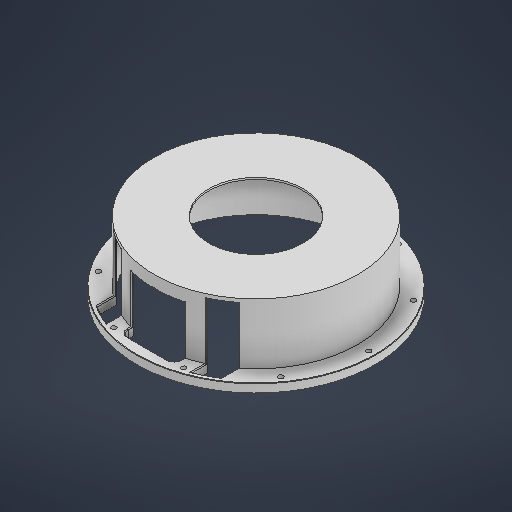
# Autodesk Inventor part: Cylinder  Segment - 01
Saved by Autodesk Inventor 2025 (Build 290162000, 162)
## iProperties
Created: 2024-04-11
Part Number: Cylinder  Segment - 01
Material: Generic
Document SubType Name: Modeling
Designer: Thienan Hoang
Density: 1 g/cm^3
Appearance: Default
Author: Thienan Hoang
Autodesk Inventor part; units mm, degrees
ref_plane "YZ Plane" through (0, 0, 0) normal (1, 0, 0) x (0, 1, 0)
ref_plane "XZ Plane" through (0, 0, 0) normal (0, 1, 0) x (-1, 0, 0)
ref_plane "XY Plane" through (0, 0, 0) normal (0, 0, 1) x (1, 0, 0)
sketch "Sketch1" plane through (0, 0, 0) normal (0, 1, 0) x (-1, 0, 0)
  circle A0 centre (0, 0) radius 135
  circle A1 centre (0, 0) radius 115
  circle A2 centre (0, 0) radius 112.0375
  circle A3 centre (0, 0) radius 9.5
  dimension "Absolute_Diameter" = 270
  dimension "Diameter_No_Outer_Lip" = 230
  dimension "Inner_Cylinder_Diameter" = 224.075
  dimension "Lip_Diameter" = 19
  constraints: 4 centre point, 4 coincident
  measures "Absolute_Diameter" diameter of A0
  measures "Diameter_No_Outer_Lip" diameter of A1
  measures "Inner_Cylinder_Diameter" diameter of A2
  measures "Lip_Diameter" diameter of A3
extrude "Extrusion1" add sketch "Sketch1" along normal blind 10 contours A0
extrude "Extrusion2" add sketch "Sketch1" along normal blind 75 contours A1
sketch "Sketch2" plane through (0, 75, 0) normal (0, 1, 0) x (1, 0, 0)
  circle A0 centre (0, 0) radius 115
  circle A1 centre (0, 0) radius 53.125
  dimension "Lip_Diameter_Out" = 230
  dimension "Inner_Lip_Diameter" = 106.25
  constraints: 2 centre point, 1 coincident
  measures "Lip_Diameter_Out" diameter of A0
  measures "Inner_Lip_Diameter" diameter of A1
extrude "Extrusion7" add sketch "Sketch2" against normal blind 5
chamfer "Chamfer1" distance 0.5 angle 45 2 edges at (115, 75, 0) (-53.125, 75, 0)
chamfer "Chamfer2" distance 0.5 angle 45 3 edges at (135, 10, 0) (135, 0, 0) (112.0375, 0, 0)
sketch "Sketch3" plane through (0, 10, 0) normal (0, 1, 0) x (1, 0, 0)
  circle A0 centre (0, 0) radius 127.5
  circle A1 centre (-127.5, 0) radius 2.75
  circle A2 centre (-103.1497, -74.9426) radius 2.75
  circle A3 centre (-39.3997, -121.2597) radius 2.75
  circle A4 centre (39.3997, -121.2597) radius 2.75
  circle A5 centre (103.1497, -74.9426) radius 2.75
  circle A6 centre (127.5, 0) radius 2.75
  circle A7 centre (103.1497, 74.9426) radius 2.75
  circle A8 centre (39.3997, 121.2597) radius 2.75
  circle A9 centre (-39.3997, 121.2597) radius 2.75
  circle A10 centre (-103.1497, 74.9426) radius 2.75
  dimension "d27" = 255
  dimension "d28" = 5.5
  dimension "d31" = 360
  constraints: 10 centre point, 1 coincident, 1 horizontal alignment, 23 other
  measures "d28" diameter of A1
extrude "Extrusion8" cut sketch "Sketch3" against normal blind 10 contours A0 A6 | A0 A6 | A7 A0 | A0 A7 | A5 A0 | A0 A5 | A8 A0 | A0 A8 | A4 A0 | A0 A4 | A9 A0 | A0 A9 | A3 A0 | A0 A3 | A10 A0 | A0 A10 | A2 A0 | A0 A2 | A1 A0 | A0 A1
chamfer "Chamfer3" [suppressed]
sketch "Sketch5" plane through (0, 75, 0) normal (0, 1, 0) x (1, 0, 0)
  circle A0 centre (0, 0) radius 39.5
  circle A1 centre (0, 0) radius 112.5375 projected
  line L0 (105.9252, 8.8939) -> (105.9252, -41.1061)
  line L1 (-117.4998, -25) -> (-117.4998, 25)
  line L2 (-117.4998, 25) -> (-51.7808, 25)
  line L3 (56.808, 8.8939) -> (105.9252, 8.8939)
  line L4 (105.9252, -41.1061) -> (40.2062, -41.1061)
  line L5 (-51.7808, -25) -> (-117.4998, -25)
  arc A2 (-51.7808, -25) -> (40.2062, -41.1061) centre (0, 0) ccw
  arc A3 (56.808, 8.8939) -> (-51.7808, 25) centre (0, 0) ccw
  dimension "d54" = 50
  dimension "d97" = 65.719
  dimension "d98" = 65.719
  dimension "d99" = 57.5
  dimension "d100" = 57.5
  dimension "d101" = 50
  dimension "d102" = 50
  dimension "d103" = 52.6842
  dimension "d104" = 223.425
  constraints: 12 end point, 5 parallel, 4 point on circle, 3 centre point, 2 coincident, 2 horizontal, 2 perpendicular
  measures "d54" distance of L0.start L0.end
  measures "d97" distance of L5.start L1.start
  measures "d98" distance of L0.end L4.end
  measures "d99" radius of A2
  measures "d100" radius of A3
  measures "d101" distance of L1.start L1.end
  measures "d102" distance of L5.start L2.end
  measures "d103" distance of L4.end L3.start
  measures "d104" distance between parallel lines of L0 L1
extrude "Extrusion9" [suppressed]
sketch "Sketch6" plane through (0, 75, 0) normal (0, -1, 0) x (1, 0, 0)
  line L0 (111.7125, -22) -> (-111.7125, -22)
  line L1 (-111.7125, -22) -> (-111.7125, 22)
  line L2 (-111.7125, 22) -> (111.7125, 22)
  line L3 (111.7125, 22) -> (111.7125, -22)
  line L4 (111.7125, -22) -> (-111.7125, 22) construction
  line L5 (-111.7125, -22) -> (111.7125, 22) construction
  line L6 (139.9625, -19.625) -> (86.4625, -19.625)
  line L7 (83.4625, -16.625) -> (83.4625, 16.625)
  line L8 (86.4625, 19.625) -> (139.9625, 19.625)
  line L9 (139.9625, 19.625) -> (139.9625, -19.625)
  line L10 (139.9625, -19.625) -> (83.4625, 19.625) construction
  line L11 (83.4625, -19.625) -> (139.9625, 19.625) construction
  line L12 (-86.4625, -19.625) -> (-139.9625, -19.625)
  line L13 (-139.9625, -19.625) -> (-139.9625, 19.625)
  line L14 (-139.9625, 19.625) -> (-86.4625, 19.625)
  line L15 (-83.4625, 16.625) -> (-83.4625, -16.625)
  line L16 (-83.4625, -19.625) -> (-139.9625, 19.625) construction
  line L17 (-139.9625, -19.625) -> (-83.4625, 19.625) construction
  arc A0 (-86.4625, -19.625) -> (-83.4625, -16.625) centre (-86.4625, -16.625) ccw
  arc A1 (-83.4625, 16.625) -> (-86.4625, 19.625) centre (-86.4625, 16.625) ccw
  arc A2 (83.4625, -16.625) -> (86.4625, -19.625) centre (86.4625, -16.625) ccw
  arc A3 (86.4625, 19.625) -> (83.4625, 16.625) centre (86.4625, 16.625) ccw
  point P0 (0, 0)
  point P1 (111.7125, 0)
  point P2 (-111.7125, 0)
  dimension "d58" = 234.5
  dimension "d59" = 44
  dimension "d60" = 56.5
  dimension "d61" = 39.25
  dimension "d62" = 56.5
  dimension "d63" = 39.25
  dimension "d64" = 3
  constraints: 36 end point, 8 midpoint, 8 point on circle, 8 point on line, 8 tangent, 6 parallel, 4 centre point, 3 equal radius, 3 horizontal, 3 perpendicular
  measures "d59" distance of L0.end L1.end
  measures "d60" distance of L10.end L8.end
  measures "d61" distance of L11.start L10.end
  measures "d62" distance of L13.end L17.end
  measures "d63" distance of L12.end L13.end
  measures "d64" radius of A0
extrude "Extrusion10" [suppressed]
sketch "Sketch8" plane through (0, 95, 0) normal (0, 1, 0) x (1, 0, 0)
  line L0 (-92.7125, 11) -> (92.7125, 11)
  line L1 (92.7125, 11) -> (92.7125, -11)
  line L2 (92.7125, -11) -> (-92.7125, -11)
  line L3 (-92.7125, -11) -> (-92.7125, 11)
  line L4 (-92.7125, 11) -> (92.7125, -11) construction
  line L5 (92.7125, 11) -> (-92.7125, -11) construction
  circle A0 centre (-92.7125, 11) radius 3.75
  circle A1 centre (-92.7125, -11) radius 3.75
  circle A2 centre (92.7125, 11) radius 3.75
  circle A3 centre (92.7125, -11) radius 3.75
  point P0 (0, 0)
  dimension "d69" = 197
  dimension "d70" = 6.35
  dimension "d71" = 4.5
  dimension "d72" = 7.5
  dimension "d73" = 7.5
  dimension "d74" = 7.5
  constraints: 12 end point, 4 centre point, 4 coincident, 2 midpoint, 2 parallel, 1 horizontal, 1 perpendicular
  measures "d72" diameter of A1
  measures "d73" diameter of A2
  measures "d74" diameter of A3
hole "Hole2" [suppressed]
hole "Hole3" [suppressed]
chamfer "Chamfer4" [suppressed]
fillet "Fillet1" [suppressed]
fillet "Fillet2" [suppressed]
chamfer "Chamfer5" [suppressed]
sketch "Sketch9" plane through (0, 95, 0) normal (0, 1, 0) x (1, 0, 0)
  line L0 (-68.2625, 6.35) -> (-65.0875, 6.35)
  line L1 (-65.0875, 6.35) -> (-65.0875, -6.35)
  line L2 (-65.0875, -6.35) -> (-68.2625, -6.35)
  line L3 (-68.2625, -6.35) -> (-68.2625, 6.35)
  line L4 (-68.2625, 6.35) -> (-65.0875, -6.35) construction
  line L5 (-65.0875, 6.35) -> (-68.2625, -6.35) construction
  line L6 (-68.2625, -6.35) -> (-66.675, -10.3402)
  line L7 (-66.675, -10.3402) -> (-65.0875, -6.35)
  point P0 (0, 0)
  point P1 (-66.675, 0)
  constraints: 16 end point, 2 midpoint, 2 parallel, 1 horizontal, 1 perpendicular
extrude "Extrusion11" [suppressed]
sketch "Sketch12" plane through (0, 75, 0) normal (0, 1, 0) x (1, 0, 0)
  circle A0 centre (0, 0) radius 40
  circle A1 centre (40, 0) radius 1.25
  circle A2 centre (28.2843, 28.2843) radius 1.25
  circle A3 centre (0, 40) radius 1.25
  circle A4 centre (-28.2843, 28.2843) radius 1.25
  circle A5 centre (-40, 0) radius 1.25
  circle A6 centre (-28.2843, -28.2843) radius 1.25
  circle A7 centre (0, -40) radius 1.25
  circle A8 centre (28.2843, -28.2843) radius 1.25
  dimension "d115" = 80
  dimension "d116" = 2.5
  dimension "d119" = 360
  constraints: 8 centre point, 1 coincident, 1 horizontal alignment, 19 other
  measures "d116" diameter of A1
sketch "Sketch13" plane through (0, 0, 0) normal (0, 0, 1) x (1, 0, 0)
  circle A0 centre (0, 45) radius 20.625
  line L0 (134.5, 0) -> (-134.5, 0) projected
  point P0 (0, 0)
  dimension "d128" = 41.25
  dimension "d129" = 45
  constraints: 1 centre point
  measures "d128" diameter of A0
  measures "d129" distance from line of L0 A0.centre
extrude "Extrusion14" cut sketch "Sketch13" along normal through all
extrude "Extrusion15" [suppressed]
sketch "Sketch14" plane through (0, 10, 0) normal (0, 1, 0) x (1, 0, 0)
  circle A0 centre (0, 0) radius 121.0576
  line L0 (-28, -171.0576) -> (28, -171.0576)
  line L1 (28, -171.0576) -> (28, -71.0576)
  line L2 (28, -71.0576) -> (-28, -71.0576)
  line L3 (-28, -71.0576) -> (-28, -171.0576)
  line L4 (-28, -171.0576) -> (28, -71.0576) construction
  line L5 (28, -171.0576) -> (-28, -71.0576) construction
  point P0 (0, -121.0576)
  dimension "d145" = 242.1153
  dimension "d146" = 56
  dimension "d147" = 100
  constraints: 12 end point, 2 midpoint, 2 parallel, 1 horizontal, 1 perpendicular, 1 vertical alignment, 2 other
  measures "d146" distance of L2.end L1.end
  measures "d147" distance of L1.end L0.end
extrude "Extrusion18" cut sketch "Sketch14" along normal blind 55 contours L3 L2 L1 A0 | A0 L1 L0 L3 picked at (0, -87.7243)
sketch "Sketch15" plane through (0, 0, 0) normal (0, -1, 0) x (1, 0, 0)
  circle A0 centre (0, 0) radius 104.7875
  line L0 (22, 122.501) -> (-22, 122.501)
  line L1 (30, 122.501) -> (74, 122.501) construction
  line L2 (30, 114.501) -> (30, 100.4013)
  line L3 (-30, 114.501) -> (-30, 100.4013)
  circle A1 centre (0, 0) radius 53.625 projected
  arc A2 (30, 114.501) -> (22, 122.501) centre (22, 114.501) ccw
  arc A3 (-22, 122.501) -> (-30, 114.501) centre (-22, 114.501) ccw
  point P0 (-30, 122.501)
  point P1 (0, 122.501)
  dimension "d151" = 180
  dimension "d152" = 122.501
  dimension "d153" = 51.1625
  dimension "d154" = 30
  dimension "d155" = 8
  dimension "d159" = 44
  constraints: 8 end point, 6 point on circle, 4 point on line, 4 tangent, 3 centre point, 2 horizontal, 1 coincident, 1 collinear, 1 equal radius, 1 midpoint, 1 parallel, 1 vertical, 1 vertical alignment
  measures "d151" angle of L0 L1
  measures "d152" distance from line of A0.centre L0
  measures "d153" radial gap between concentric circles of A1 A0
  measures "d154" distance from line of point (0, 0) L2
  measures "d155" radius of A2
  measures "d159" distance of L0.start L0.end
extrude "Extrusion19" cut sketch "Sketch15" against normal up to surface (65 mm away) contours A0 L3 A3 L0 A2 L2
sketch "Sketch16" plane through (0, 0, 0) normal (0, -1, 0) x (1, 0, 0)
  circle A0 centre (0, 0) radius 108
  line L0 (-48.125, 96.685) -> (-48.125, 120.7642)
  line L1 (-30, 108.4652) -> (-30, 114.501) projected
  circle A1 centre (0, 0) radius 130
  line L2 (-70.125, 82.137) -> (-70.125, 109.4645)
  line L3 (-70.125, 82.137) -> (-48.125, 82.137)
  line L4 (-48.125, 82.137) -> (-48.125, 74.6125)
  line L5 (-48.125, 74.6125) -> (-70.125, 74.6125)
  line L6 (-70.125, 74.6125) -> (-70.125, 82.137)
  line L7 (-48.125, 96.685) -> (-48.125, 82.137)
  line L8 (48.125, 96.685) -> (48.125, 120.7642)
  line L9 (30, 114.501) -> (30, 108.4652) projected
  line L10 (70.125, 82.137) -> (70.125, 109.4645)
  circle A2 centre (0, 0) radius 130
  point P0 (70.125, 109.4645)
  dimension "d160" = 18.125
  dimension "d163" = 18.125
  dimension "d164" = 22
  dimension "d165" = 22
  dimension "d166" = 260
  dimension "d167" = 260
  dimension "d170" = 216
  dimension "d181" = 48.125
  constraints: 18 end point, 8 point on circle, 4 parallel, 3 centre point, 3 coincident, 1 collinear, 1 horizontal, 1 perpendicular, 1 vertical
  measures "d160" distance between parallel lines of L1 L0
  measures "d163" distance between parallel lines of L8 L9
  measures "d164" distance of L4.end L5.end
  measures "d165" distance between parallel lines of L8 L10
  measures "d166" diameter of A2
  measures "d167" diameter of A1
  measures "d170" diameter of A0
  measures "d181" distance from line of point (0, 0) L8
extrude "Extrusion21" cut sketch "Sketch16" against normal blind 75 contours A0 L8 A1 L10 | L2 A1 L0 A0
sketch "Sketch17" plane through (0, 75, 0) normal (0, 1, 0) x (1, 0, 0)
  circle A0 centre (0, 0) radius 115
  line L0 (-51.125, -51.25) -> (-26.125, -51.25)
  line L1 (-26.125, -51.25) -> (-26.125, -96.25)
  line L2 (-26.125, -96.25) -> (-51.125, -96.25)
  line L3 (-51.125, -96.25) -> (-51.125, -51.25)
  line L4 (-51.125, -51.25) -> (-26.125, -96.25) construction
  line L5 (-26.125, -51.25) -> (-51.125, -96.25) construction
  line L6 (-48.125, -104.4461) -> (-48.125, -120.7642) projected
  point P0 (-38.625, -73.75)
  dimension "d171" = 25
  dimension "d172" = 45
  dimension "d173" = 3
  dimension "d174" = 96.25
  constraints: 12 end point, 2 midpoint, 2 parallel, 1 coincident, 1 horizontal, 1 perpendicular, 2 other
  measures "d171" distance of L1.end L2.end
  measures "d172" distance of L0.end L1.end
  measures "d173" distance between parallel lines of L3 L6
  measures "d174" distance from line of point (0, 0) L2
extrude "Extrusion22" cut sketch "Sketch17" against normal blind 10 contours L0 L1 L2 L3
sketch "Sketch18" plane through (0, 75, 0) normal (0, 1, 0) x (1, 0, 0)
  circle A0 centre (0, 0) radius 115
  circle A1 centre (0, 0) radius 53.3681
  dimension "d182" = 230
  constraints: 2 centre point, 2 coincident
  measures "d182" diameter of A0
extrude "Extrusion23" add sketch "Sketch18" along normal mid plane 1
sketch "Sketch20" plane through (0, 75.5, 0) normal (0, 1, 0) x (1, 0, 0)
  circle A0 centre (0, 0) radius 115
  circle A1 centre (0, 0) radius 53.3681
  constraints: 2 centre point, 1 coincident
extrude "Extrusion25" add sketch "Sketch20" along normal blind 3
sketch "Sketch19" plane through (0, 70, 0) normal (0, -1, 0) x (1, 0, 0)
  circle A0 centre (0, 0) radius 112.0375
  constraints: 1 centre point, 1 coincident
extrude "Extrusion24" cut sketch "Sketch19" against normal blind 6.5
chamfer "Chamfer8" distance 1 angle 45 11 edges at (-70.125, 10, 100.305) (-59.3943, 10, 115.6387) (-48.125, 10, 112.6051) (-27.6569, 10, 120.1579) (-30, 10, 112.7595) (0, 10, 122.501) (27.6569, 10, 120.1579) (30, 10, 112.7595) (48.125, 10, 112.6051) (59.3943, 10, 115.6387) (70.125, 10, 100.305)
fillet "Fillet3" radius 1 22 edges at (-30, 37.5, 111.018) (-30, 9.5, 111.018) (-30, 32.75, 107.9463) (-48.125, 42.25, 104.4461) (-48.125, 9.5, 104.4461) (-70.125, 9.5, 91.1454) (-70.125, 42.25, 91.1454) (-70.125, 35.25, 87.3778) (-70.125, 72.25, 87.3778) (-48.125, 72.25, 101.175) (-48.125, 35.25, 101.175) (30, 32.75, 107.9463) (30, 9.5, 111.018) (30, 37.5, 111.018) (48.125, 9.5, 104.4461) (48.125, 42.25, 104.4461) (48.125, 72.25, 101.175) (48.125, 35.25, 101.175) (70.125, 9.5, 91.1454) (70.125, 42.25, 91.1454) (70.125, 35.25, 87.3778) (70.125, 72.25, 87.3778)
body "Solid1"
